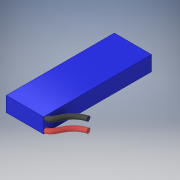
# Autodesk Inventor part: Battery
Saved by Autodesk Inventor 2019.2 (Build 232265000, 265)
## iProperties
Created: 2019-06-09
Part Number: Battery
Material: Generic
Document SubType Name: Modeling
Designer: Johansson
Density: 1 g/cm^3
Appearance: Default
Author: Johansson
Autodesk Inventor part; units mm, degrees
ref_plane "YZ Plane" through (0, 0, 0) normal (1, 0, 0) x (0, 1, 0)
ref_plane "XZ Plane" through (0, 0, 0) normal (0, 1, 0) x (-1, 0, 0)
ref_plane "XY Plane" through (0, 0, 0) normal (0, 0, 1) x (1, 0, 0)
sketch "Sketch1" plane through (0, 0, 0) normal (0, 1, 0) x (-1, 0, 0)
  line L0 (-25, 72.5) -> (25, 72.5)
  line L1 (25, 72.5) -> (25, -72.5)
  line L2 (25, -72.5) -> (-25, -72.5)
  line L3 (-25, -72.5) -> (-25, 72.5)
  line L4 (-25, 72.5) -> (25, -72.5) construction
  line L5 (25, 72.5) -> (-25, -72.5) construction
  point P0 (0, 0)
  dimension "d0" = 145
  dimension "d1" = 50
  constraints: 12 end point, 2 midpoint, 2 parallel, 1 horizontal, 1 perpendicular
  measures "d0" distance of L0.end L1.end
  measures "d1" distance of L1.end L2.end
extrude "Extrusion1" add sketch "Sketch1" along normal blind 20
sketch "Sketch2" plane through (25, 0, 72.5) normal (1, 0, 0) x (0, 0, -1)
  circle A0 centre (3, 17) radius 3
  circle A1 centre (3, 3) radius 3
  line L0 (0, 20) -> (145, 20) projected
  line L1 (0, 0) -> (0, 20) projected
  line L2 (145, 0) -> (0, 0) projected
  point P0 (72.5, 0)
  dimension "d4" = 6
  constraints: 4 tangent, 2 centre point, 1 equal radius
  measures "d4" diameter of A1
sketch "Sketch3" plane through (0, 20, 0) normal (0, 1, 0) x (1, 0, 0)
  line L0 (25, -72.5) -> (25, 72.5) projected
  spline S0 degree 3 poles (25, -69.5942) (35.7518, -68.7484) (31.9339, -48.3248) (54.1894, -41.5188) knots 0 0 0 0 1 1 1 1
  point P0 (0, 0)
  point P1 (30.8131, -66.0232)
  point P2 (36.5071, -55.5607)
  constraints: 1 point on line, 4 other
sweep "Sweep1" add profiles "Sketch2" path "Sketch3" path curves S0 contours A0
sweep "Sweep2" add profiles "Sketch2" path "Sketch3" separate body path curves S0 contours A1
equation "\"d0\" = L_Battery"
equation "\"d1\" = W_Battery"
equation "\"d2\" = H_Battery"
equation "\"DO_BLDC\" = 63"
equation "\"WO_BLDC\" = 64"
equation "\"D_Shaft_BLDC\" = 8"
equation "\"D_Hole_BLDC\" = 45.5"
equation "\"W_Wall\" = 8"
equation "\"T_WheelToShaft\" = 0.3"
equation "\"W_WheelOuter\" = 25"
equation "\"W_Battery\" = 50"
equation "\"L_Battery\" = 145"
equation "\"H_Battery\" = 20"
body "Solid1"
body "Solid2"
